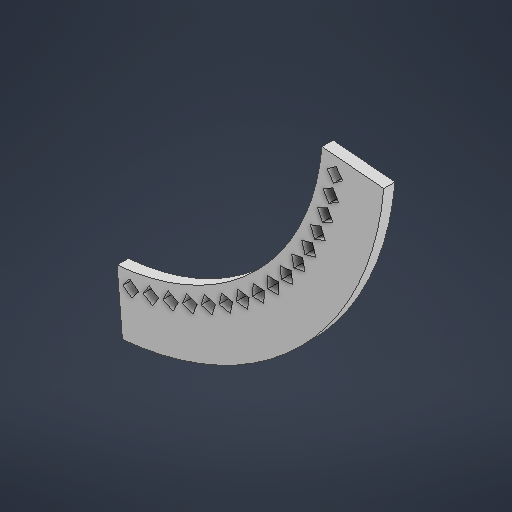
# Autodesk Inventor part: shim_cartridge
Saved by Autodesk Inventor 2026.1 (Build 301233020, 233B)
## iProperties
Created: 2024-04-08
Part Number: shim_cartridge
Material: Generic
Document SubType Name: Modeling
Designer: Joshua Harper
Density: 1 g/cm^3
Appearance: Default
Author: Joshua Harper
Autodesk Inventor part; units mm, degrees
ref_plane "YZ Plane" through (0, 0, 0) normal (1, 0, 0) x (0, 1, 0)
ref_plane "XZ Plane" through (0, 0, 0) normal (0, 1, 0) x (-1, 0, 0)
ref_plane "XY Plane" through (0, 0, 0) normal (0, 0, 1) x (1, 0, 0)
sketch "Sketch1" plane through (0, 0, 0) normal (0, 0, 1) x (1, 0, 0)
  arc A0 (6.6674, -76.2089) -> (76.2089, -6.6674) centre (0, 0) ccw
  arc A1 (5.2293, -59.7717) -> (59.7717, -5.2293) centre (0, 0) ccw
  line L0 (0, 0) -> (0, 0) construction
  line L1 (0, 0) -> (0, -128.2305) construction
  line L2 (0, 0) -> (64.2859, 0) construction
  line L3 (59.7717, -5.2293) -> (76.2089, -6.6674)
  line L4 (5.2293, -59.7717) -> (6.6674, -76.2089)
  line L5 (0, 0) -> (6.6674, -76.2089) construction
  line L6 (0, 0) -> (76.2089, -6.6674) construction
  dimension "d0" = 153
  dimension "d1" = 120
  dimension "d59" = 5
  dimension "d61" = 5
  constraints: 14 end point, 5 coincident, 5 point on circle, 2 centre point, 2 collinear, 2 vertical, 1 horizontal
  measures "d0" diameter of A0
  measures "d1" diameter of A1
  measures "d59" angle of L5 L1
  measures "d61" angle of L2 L6
extrude "Extrusion1" add sketch "Sketch1" along normal blind 3
sketch "Sketch5" plane through (0, 0, 3) normal (0, 0, 1) x (1, 0, 0)
  line L0 (8.6118, -61.2765) -> (11.0078, -63.0819)
  line L1 (11.0078, -63.0819) -> (9.2023, -65.4778)
  line L2 (9.2023, -65.4778) -> (6.8064, -63.6724)
  line L3 (6.8064, -63.6724) -> (8.6118, -61.2765)
  line L4 (0, 0) -> (9.2023, -65.4778) construction
  line L5 (11.0078, -63.0819) -> (6.8064, -63.6724) construction
  line L6 (0, 0) -> (0, -125.3413) construction
  line L7 (12.1837, -62.8654) -> (13.7793, -60.325)
  line L8 (13.7793, -60.325) -> (16.3198, -61.9206)
  line L9 (16.3198, -61.9206) -> (14.7241, -64.4611)
  line L10 (14.7241, -64.4611) -> (12.1837, -62.8654)
  line L11 (17.4731, -61.6051) -> (18.8475, -58.9385)
  line L12 (18.8475, -58.9385) -> (21.5141, -60.3129)
  line L13 (21.5141, -60.3129) -> (20.1397, -62.9795)
  line L14 (20.1397, -62.9795) -> (17.4731, -61.6051)
  line L15 (22.6365, -59.9007) -> (23.7797, -57.127)
  line L16 (23.7797, -57.127) -> (26.5533, -58.2702)
  line L17 (26.5533, -58.2702) -> (25.4101, -61.0439)
  line L18 (25.4101, -61.0439) -> (22.6365, -59.9007)
  line L19 (27.6367, -57.7643) -> (28.5405, -54.9037)
  line L20 (28.5405, -54.9037) -> (31.4011, -55.8075)
  line L21 (31.4011, -55.8075) -> (30.4973, -58.6681)
  line L22 (30.4973, -58.6681) -> (27.6367, -57.7643)
  line L23 (32.4376, -55.2114) -> (33.0954, -52.2844)
  line L24 (33.0954, -52.2844) -> (36.0224, -52.9423)
  line L25 (36.0224, -52.9423) -> (35.3646, -55.8693)
  line L26 (35.3646, -55.8693) -> (32.4376, -55.2114)
  line L27 (37.0046, -52.2605) -> (37.4118, -49.2882)
  line L28 (37.4118, -49.2882) -> (40.384, -49.6954)
  line L29 (40.384, -49.6954) -> (39.9769, -52.6676)
  line L30 (39.9769, -52.6676) -> (37.0046, -52.2605)
  line L31 (41.3049, -48.9327) -> (41.4584, -45.9366)
  line L32 (41.4584, -45.9366) -> (44.4545, -46.0901)
  line L33 (44.4545, -46.0901) -> (44.3009, -49.0862)
  line L34 (44.3009, -49.0862) -> (41.3049, -48.9327)
  line L35 (45.3073, -45.2521) -> (45.2061, -42.2538)
  line L36 (45.2061, -42.2538) -> (48.2044, -42.1526)
  line L37 (48.2044, -42.1526) -> (48.3056, -45.1509)
  line L38 (48.3056, -45.1509) -> (45.3073, -45.2521)
  line L39 (48.983, -41.2452) -> (48.6278, -38.2663)
  line L40 (48.6278, -38.2663) -> (51.6067, -37.9111)
  line L41 (51.6067, -37.9111) -> (51.9619, -40.89)
  line L42 (51.9619, -40.89) -> (48.983, -41.2452)
  line L43 (52.3055, -36.9409) -> (51.6989, -34.0029)
  line L44 (51.6989, -34.0029) -> (54.6369, -33.3962)
  line L45 (54.6369, -33.3962) -> (55.2436, -36.3343)
  line L46 (55.2436, -36.3343) -> (52.3055, -36.9409)
  line L47 (55.2509, -32.3703) -> (54.3972, -29.4943)
  line L48 (54.3972, -29.4943) -> (57.2732, -28.6406)
  line L49 (57.2732, -28.6406) -> (58.1269, -31.5166)
  line L50 (58.1269, -31.5166) -> (55.2509, -32.3703)
  line L51 (57.7979, -27.5662) -> (56.7033, -24.7731)
  line L52 (56.7033, -24.7731) -> (59.4965, -23.6784)
  line L53 (59.4965, -23.6784) -> (60.5911, -26.4716)
  line L54 (60.5911, -26.4716) -> (57.7979, -27.5662)
  line L55 (59.9282, -22.5634) -> (58.6006, -19.8732)
  line L56 (58.6006, -19.8732) -> (61.2908, -18.5456)
  line L57 (61.2908, -18.5456) -> (62.6185, -21.2358)
  line L58 (62.6185, -21.2358) -> (59.9282, -22.5634)
  line L59 (61.6264, -17.3979) -> (60.0753, -14.83)
  line L60 (60.0753, -14.83) -> (62.6432, -13.279)
  line L61 (62.6432, -13.279) -> (64.1943, -15.8469)
  line L62 (64.1943, -15.8469) -> (61.6264, -17.3979)
  line L63 (62.8802, -12.107) -> (61.1169, -9.68)
  line L64 (61.1169, -9.68) -> (63.5439, -7.9166)
  line L65 (63.5439, -7.9166) -> (65.3073, -10.3437)
  line L66 (65.3073, -10.3437) -> (62.8802, -12.107)
  line L67 (61.1169, -9.68) -> (65.3073, -10.3437) construction
  point P0 (8.9071, -63.3772)
  dimension "d43" = 3
  dimension "d44" = 64
  dimension "d45" = 8
  dimension "d48" = 73
  dimension "d58" = 73
  constraints: 136 end point, 3 perpendicular, 2 parallel, 2 point on line, 1 midpoint, 1 vertical, 121 other
  measures "d43" distance of L2.end L0.start
  measures "d44" distance of point (8.907, -63.377) L4.start
  measures "d45" angle of L4 L6
  measures "d58" angle of L67 L4
extrude "Extrusion5" cut sketch "Sketch5" against normal through all
equation "\"d61\" = d59"
body "Solid1"
